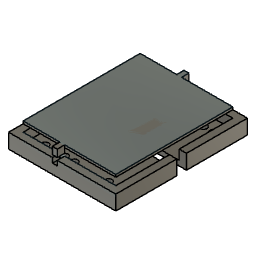
caja v2 (Autodesk Fusion 360 design; units mm, degrees)
Autodesk Fusion 360 part; units mm, degrees
sketch "Boceto1" plane through (0, 0, 0) normal (0, 0, 1) x (1, 0, 0)
  line L0 (0, 0) -> (220, 0)
  line L1 (220, 0) -> (220, -250)
  line L2 (220, -250) -> (0, -250)
  line L3 (0, -250) -> (0, 0)
  dimension "d1" = 220
  constraint horizontal L0
  constraint vertical L1
  constraint horizontal L2
  constraint vertical L3
  constraint coincident L0.start L3.end
  measures "d1" distance of L0.start L0.end
extrude "Extruir1" add sketch "Boceto1" along normal blind 30 makes body 1
shell "Vaciado1" thickness 15 removed faces 2 at (73.3333, -83.3333, 30) at (73.3333, -83.3333, 0) on bodies 1
sketch "Boceto2" plane through (0, 0, 0) normal (0, 0, 1) x (1, 0, 0)
  line L0 (205, -235) -> (15, -235)
  line L1 (15, -235) -> (15, -15)
  line L2 (15, -15) -> (205, -15)
  line L3 (205, -15) -> (205, -235)
  constraint horizontal L0
  constraint vertical L1
  constraint horizontal L2
  constraint vertical L3
extrude "Extruir2" add sketch "Boceto2" along normal blind 10 bodies 1
sketch "Boceto3" plane through (0, 0, 10) normal (0, 0, 1) x (-1, 0, 0)
  line L0 (-205, 15) -> (-15, 15)
  line L1 (-15, 15) -> (-15, 235)
  line L2 (-15, 235) -> (-205, 235)
  line L3 (-205, 235) -> (-205, 15)
  circle A0 centre (-40, 40) radius 7.0711
  circle A1 centre (-60, 40) radius 7.0711
  circle A2 centre (-80, 40) radius 7.0711
  circle A3 centre (-190, 40) radius 7.0711
  circle A4 centre (-170, 40) radius 7.0711
  circle A5 centre (-40, 215) radius 7.0711
  circle A6 centre (-60, 215) radius 7.0711
  circle A7 centre (-80, 215) radius 7.0711
  circle A8 centre (-100, 215) radius 7.0711
  circle A9 centre (-170, 215) radius 7.0711
extrude "Extruir3" cut sketch "Boceto3" along normal blind 10 and the other way blind 30 contours A0 | A1 | A2 | A3 | A4 | A5 | A6 | A7 | A8 | A9 bodies 1
sketch "Boceto4" plane through (0, 0, 10) normal (0, 0, 1) x (-1, 0, 0)
  circle A0 centre (-80, 215) radius 7.0711
  circle A1 centre (-170, 40) radius 7.0711
  circle A2 centre (-40, 40) radius 7.0711
  circle A3 centre (-190, 40) radius 7.0711
  circle A4 centre (-100, 215) radius 7.0711
  circle A5 centre (-60, 215) radius 7.0711
  circle A6 centre (-80, 40) radius 7.0711
  circle A7 centre (-60, 40) radius 7.0711
  circle A8 centre (-40, 215) radius 7.0711
  circle A9 centre (-170, 215) radius 7.0711
  line L0 (-205, 15) -> (-15, 15)
  line L1 (-15, 15) -> (-15, 235)
  line L2 (-15, 235) -> (-205, 235)
  line L3 (-205, 235) -> (-205, 15)
  line L4 (0, 125) -> (-220, 125)
  line L5 (0, 0) -> (-111, 0)
  line L6 (-111, 0) -> (-111, 235)
  constraint perpendicular L3 L4
  constraint coincident L5.start origin
  constraint parallel L0 L5
  constraint coincident L2 L6.end
  constraint perpendicular L2 L6
split "Dividir1" by curves path "Boceto4" along L4 bodies 1 makes body 2 at (106.8428, -152.6496, 0)
sketch "Boceto5" plane through (0, -235, 0) normal (0, 1, 0) x (-1, 0, 0)
  line L0 (-205, 10) -> (-15, 10)
  line L1 (-15, 10) -> (-15, 30)
  line L2 (-15, 30) -> (-205, 30)
  line L3 (-205, 30) -> (-205, 10)
move_body "Desplazar1" bodies 1 to x (1, 0, 0) y (0, 1, 0) z (0, 0, 1) at (0, 20, 0)
sketch "Boceto6" plane through (0, 0, 10) normal (0, 0, 1) x (-1, 0, 0)
  line L0 (-15, 105) -> (-205, 105)
  line L1 (-205, 105) -> (-205, -5)
  line L2 (-205, -5) -> (-15, -5)
  line L3 (-15, -5) -> (-15, 105)
  circle A0 centre (-60, 20) radius 7.0711
  circle A1 centre (-80, 20) radius 7.0711
  circle A2 centre (-190, 20) radius 7.0711
  circle A3 centre (-40, 20) radius 7.0711
  circle A4 centre (-170, 20) radius 7.0711
  circle A5 centre (-80, 100) radius 10
  circle A6 centre (-150, 100) radius 10
extrude "Extruir4" cut sketch "Boceto6" along normal blind 40 and the other way blind 20 contours L0 A5 | L0 A6 picked at (-77.3805, 95.2901) picked at (-148.9394, 96.4227) bodies 1
sketch "Boceto7" plane through (0, 0, 10) normal (0, 0, 1) x (-1, 0, 0)
  line L0 (-205, 125) -> (-15, 125)
  line L1 (-15, 125) -> (-15, 235)
  line L2 (-15, 235) -> (-205, 235)
  line L3 (-205, 235) -> (-205, 125)
  circle A0 centre (-80, 215) radius 7.0711
  circle A1 centre (-100, 215) radius 7.0711
  circle A2 centre (-60, 215) radius 7.0711
  circle A3 centre (-40, 215) radius 7.0711
  circle A4 centre (-170, 215) radius 7.0711
  circle A5 centre (-150, 120) radius 9.8
  circle A6 centre (-80, 120) radius 9.8
  dimension "d16" = 19.6
  dimension "d17" = 19.6
  measures "d16" diameter of A5
  measures "d17" diameter of A6
extrude "Extruir5" add sketch "Boceto7" along normal blind 0 and the other way blind 10 contours L0 A5 | L0 A6 picked at (-150.6303, 120.1281) picked at (-81.0932, 120.255) bodies 2
sketch "Boceto8" plane through (0, 0, 0) normal (0, 0, 1) x (1, 0, 0)
  line L0 (205, -235) -> (15, -235)
  line L1 (15, -235) -> (15, 5)
  line L2 (15, 5) -> (205, 5)
  line L3 (205, 5) -> (205, -235)
  line L4 (15, 5) -> (205, 5)
  line L5 (205, 5) -> (205, -235)
  line L6 (205, -235) -> (15, -235)
  line L7 (15, -235) -> (15, 5)
  constraint horizontal L0
  constraint vertical L1
  constraint horizontal L2
  constraint vertical L3
  constraint horizontal L4
  constraint vertical L5
  constraint horizontal L6
  constraint vertical L7
extrude "Extruir6" add sketch "Boceto8" along normal blind 50 and the other way blind -45 separate body makes body 3
sketch "Boceto10" plane through (0, 0, 30) normal (0, 0, 1) x (-1, 0, 0)
  line L0 (0, 105) -> (-15, 105)
  line L1 (-15, 105) -> (-15, -5)
  line L2 (-15, -5) -> (-205, -5)
  line L3 (-205, -5) -> (-205, 105)
  line L4 (-205, 105) -> (-220, 105)
  line L5 (-220, 105) -> (-220, -20)
  line L6 (-220, -20) -> (0, -20)
  line L7 (0, -20) -> (0, 105)
  line L8 (-90, 0) -> (-100, 0)
  line L9 (-100, 0) -> (-100, -20)
  line L10 (-100, -20) -> (-90, -20)
  line L11 (-90, -20) -> (-90, 0)
  constraint horizontal L8
  constraint vertical L9
  constraint horizontal L10
  constraint vertical L11
  constraint coincident L6 L9.end
extrude "Extruir7" cut sketch "Boceto10" along normal blind 55 and the other way blind 15 contours L2 L6 L9 L10 L11 bodies 1
sketch "Boceto11" plane through (0, 0, 0) normal (0, 0, 1) x (1, 0, 0)
  line L0 (100, 20) -> (90, 20)
  line L1 (90, 20) -> (90, 5)
  line L2 (90, 5) -> (100, 5)
  line L3 (100, 5) -> (100, 20)
  constraint horizontal L0
  constraint vertical L1
  constraint horizontal L2
  constraint vertical L3
extrude "Extruir8" add sketch "Boceto11" along normal blind 50 and the other way blind -35 bodies 3
sketch "Boceto12" plane through (0, 0, 50) normal (0, 0, 1) x (-1, 0, 0)
  line L0 (-15, 235) -> (-205, 235)
  line L1 (-205, 235) -> (-205, -5)
  line L2 (-205, -5) -> (-100, -5)
  line L3 (-100, -5) -> (-100, -20)
  line L4 (-100, -20) -> (-90, -20)
  line L5 (-90, -20) -> (-90, -5)
  line L6 (-90, -5) -> (-15, -5)
  line L7 (-15, -5) -> (-15, 235)
sketch "Boceto13" plane through (0, 0, 0) normal (0, 0, 1) x (1, 0, 0)
  line L0 (90, 5) -> (90, -234.8012)
  line L1 (90, -234.8012) -> (100, -234.8012)
  line L2 (100, -234.8012) -> (100, 5)
  line L3 (100, 5) -> (90, 5)
  line L4 (100, -234.8012) -> (100, -234.8012)
  line L5 (100, -234.8012) -> (100, -250)
  line L6 (100, -250) -> (100, -250)
  line L7 (100, -250) -> (100, -234.8012)
  line L8 (100, -250) -> (90, -250)
  line L9 (90, -250) -> (90, -234.8012)
  constraint vertical L0
  constraint perpendicular L0 L1
  constraint perpendicular L1 L2
  constraint perpendicular L0 L3
  constraint vertical L5
  constraint vertical L7
  constraint perpendicular L5 L8
  constraint perpendicular L1 L9
extrude "Extruir9" cut sketch "Boceto13" along normal blind 30 and the other way blind -15 contours L1 L5 L7 L8 L9 bodies 2
sketch "Boceto14" plane through (0, 0, 15) normal (0, 0, 1) x (-1, 0, 0)
  line L0 (-100, 235) -> (-90, 235)
  line L1 (-90, 235) -> (-90, 250)
  line L2 (-90, 250) -> (-100, 250)
  line L3 (-100, 250) -> (-100, 235)
  line L4 (-90, 235) -> (-100, 235)
  line L5 (-100, 235) -> (-100, 250)
  line L6 (-100, 250) -> (-90, 250)
  line L7 (-90, 250) -> (-90, 235)
  constraint horizontal L4
  constraint vertical L5
  constraint horizontal L6
  constraint vertical L7
  constraint coincident L2.end L3.start
  constraint coincident L0.end L1.start
extrude "Extruir10" add sketch "Boceto14" along normal blind 35 and the other way blind -20 bodies 3
extrude "Extruir11" add 1 faces at (96.6667, -245, 15) along direction (0, 0, 1) blind 5 on bodies 2 bodies 2
extrude "Extruir12" add 1 faces at (93.3333, 15, 15) along direction (0, 0, 1) blind 5 on bodies 1 bodies 1
